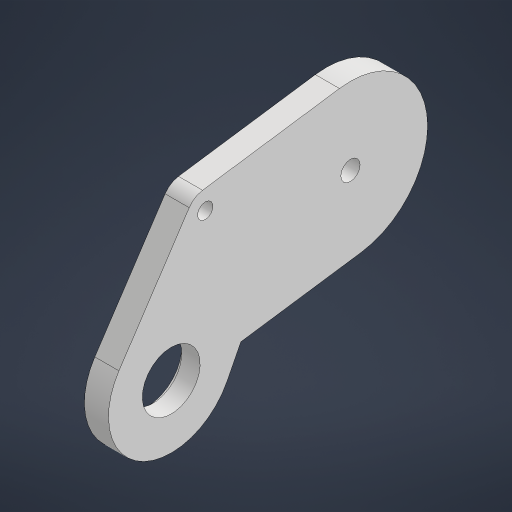
# Autodesk Inventor part: GearCover
Saved by Autodesk Inventor 2024.2 (Build 282272000, 272)
## iProperties
Created: 2023-12-29
Part Number: GearCover
Material: 一般
Document SubType Name: Modeling
Designer: Hanaoka
Density: 1 g/cm^3
Appearance: 既定
Author: Hanaoka
Autodesk Inventor part; units mm, degrees
ref_plane "YZ Plane" through (0, 0, 0) normal (1, 0, 0) x (0, 1, 0)
ref_plane "XZ Plane" through (0, 0, 0) normal (0, 1, 0) x (-1, 0, 0)
ref_plane "XY Plane" through (0, 0, 0) normal (0, 0, 1) x (1, 0, 0)
sketch "スケッチ1" plane through (0, 0, 0) normal (1, 0, 0) x (0, 1, 0)
  circle A0 centre (-9.5887, 18.586) radius 3.6
  circle A1 centre (-9.5887, 18.586) radius 3
  arc A2 (-6.0008, 24.006) -> (-12.5231, 12.786) centre (-9.5887, 18.586) ccw
  line L0 (-12.5231, 12.786) -> (-9.7122, 11.3639)
  line L1 (-9.7122, 11.3639) -> (-7.9189, -1.1361)
  line L2 (7.9189, 1.1361) -> (5.8818, 15.3361)
  line L3 (5.006, 16.7197) -> (-6.0008, 24.006)
  circle A3 centre (-9.5887, 18.586) radius 5
  circle A4 centre (-2.9179, 14.1701) radius 3
  arc A5 (5.8818, 15.3361) -> (5.006, 16.7197) centre (3.902, 15.052) ccw
  circle A6 centre (3.902, 15.052) radius 0.8
  circle A7 centre (3.902, 15.052) radius 2 construction
  circle A8 centre (-2.9179, 14.1701) radius 0.75
  line L4 (-9.5887, 18.586) -> (-2.9179, 14.1701) construction
  arc A9 (-7.9189, -1.1361) -> (7.9189, 1.1361) centre (0, 0) ccw
  circle A10 centre (0, 0) radius 1
  point P0 (5.7543, 16.2244)
  dimension "d0" = 6
  dimension "d1" = 7.2
  dimension "d2" = 6.5
  dimension "d7" = 10
  dimension "d8" = 6
  dimension "d9" = 2
  dimension "d10" = 1.6
  dimension "d11" = 4
  dimension "d12" = 1.5
  dimension "d13" = 125
  dimension "d14" = 8
  dimension "d15" = 2
  dimension "d16" = 12.5
  dimension "d17" = 14.2
  dimension "d18" = 13.2
  constraints: 11 centre point, 10 end point, 8 coincident, 7 tangent, 6 point on circle, 2 parallel, 2 point on line
  measures "d0" diameter of A1
  measures "d1" diameter of A0
  measures "d2" radius of A2
  measures "d7" diameter of A3
  measures "d8" diameter of A4
  measures "d9" radius of A5
  measures "d10" diameter of A6
  measures "d11" diameter of A7
  measures "d12" diameter of A8
  measures "d13" angle of L1 L0
  measures "d14" radius of A9
  measures "d15" diameter of A10
  measures "d16" vertical distance of L0.end L1.end
  measures "d17" vertical distance of L2.start L2.end
  measures "d18" distance of L3.start L3.end
extrude "押し出し1" add sketch "スケッチ1" along normal blind 2.5 contours A0 | L3 A5 L2 A9 L1 L0 A2 | A3 | A4 | A8
extrude "押し出し2" cut sketch "スケッチ1" along normal blind 0.6 contours A0
